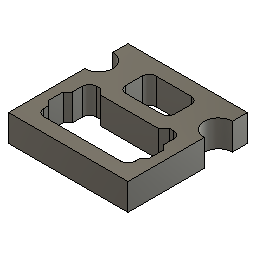
TinyNES_Foam_Top (Autodesk Fusion 360 design; units mm, degrees)
Autodesk Fusion 360 part; units mm, degrees
sketch "Sketch1" plane through (0, 0, 0) normal (0, 1, 0) x (1, 0, 0)
  line L0 (0, 0) -> (170, 0)
  line L1 (170, 0) -> (170, 170)
  line L2 (170, 170) -> (0, 170)
  line L3 (0, 170) -> (0, 0)
  line L4 (85, 170) -> (85, 128.5) construction
  line L5 (110, 107) -> (60, 107)
  line L6 (50, 117) -> (50, 140)
  line L7 (60, 150) -> (110, 150)
  line L8 (120, 140) -> (120, 117)
  line L9 (120, 107) -> (50, 150) construction
  line L10 (50, 107) -> (120, 150) construction
  arc A0 (60, 150) -> (50, 140) centre (60, 140) ccw
  arc A1 (120, 140) -> (110, 150) centre (110, 140) ccw
  arc A2 (110, 107) -> (120, 117) centre (110, 117) ccw
  arc A3 (50, 117) -> (60, 107) centre (60, 117) ccw
  line L11 (85, 128.5) -> (0, 128.5) construction
  line L12 (85, 128.5) -> (170, 128.5) construction
  arc A4 (0, 108.5) -> (0, 148.5) centre (0, 128.5) ccw
  arc A5 (170, 148.5) -> (170, 108.5) centre (170, 128.5) ccw
  line L13 (85, 0) -> (85, 53.5) construction
  line L14 (140, 20) -> (30, 20)
  line L15 (20, 30) -> (20, 87)
  line L16 (150, 87) -> (150, 30)
  line L17 (150, 20) -> (20, 87) construction
  line L18 (20, 20) -> (150, 87) construction
  arc A6 (20, 30) -> (30, 20) centre (30, 30) ccw
  arc A7 (140, 20) -> (150, 30) centre (140, 30) ccw
  line L19 (85, 53.5) -> (20, 53.5) construction
  line L20 (85, 53.5) -> (150, 53.5) construction
  line L21 (20, 53.5) -> (13.5, 53.5) construction
  line L22 (13.5, 53.5) -> (13.5, 64)
  line L23 (13.5, 53.5) -> (13.5, 43)
  line L24 (13.5, 43) -> (13.5, 36.5) construction
  line L25 (13.5, 36.5) -> (20, 36.5) construction
  line L26 (13.5, 64) -> (13.5, 70.5) construction
  line L27 (13.5, 70.5) -> (20, 70.5) construction
  line L28 (13.5, 64) -> (20, 70.5)
  line L29 (13.5, 43) -> (20, 36.5)
  line L30 (156.5, 64) -> (150, 70.5)
  line L31 (156.5, 53.5) -> (156.5, 64)
  line L32 (156.5, 53.5) -> (156.5, 43)
  line L33 (156.5, 43) -> (150, 36.5)
  line L34 (85, 53.5) -> (85, 87) construction
  line L35 (85, 128.5) -> (85, 87) construction
  line L36 (85, 87) -> (43.25, 87)
  line L37 (43.25, 87) -> (35.25, 95)
  line L38 (30, 95) -> (35.25, 95)
  line L39 (35.25, 95) -> (35.25, 87) construction
  line L40 (35.25, 87) -> (43.25, 87) construction
  line L41 (30, 95) -> (30, 85) construction
  arc A8 (30, 95) -> (20, 85) centre (30, 85) ccw
  line L42 (30, 85) -> (30, 95) construction
  line L43 (30, 85) -> (20, 85) construction
  arc A9 (150, 85) -> (140, 95) centre (140, 85) ccw
  line L44 (140, 95) -> (134.75, 95)
  line L45 (126.75, 87) -> (134.75, 95)
  line L46 (85, 87) -> (126.75, 87)
  point P0 (85, 128.5)
  point P1 (85, 53.5)
  dimension "d1" = 170
  dimension "d2" = 170
  dimension "d19" = 41.5
  dimension "d20" = 70
  dimension "d21" = 43
  dimension "d22" = 10
  dimension "d23" = 10
  dimension "d24" = 10
  dimension "d25" = 10
  dimension "d26" = 20
  dimension "d27" = 20
  dimension "d28" = 53.5
  dimension "d29" = 130
  dimension "d30" = 67
  dimension "d31" = 10
  dimension "d32" = 10
  dimension "d33" = 6.5
  dimension "d34" = 10.5
  dimension "d35" = 10.5
  dimension "d36" = 6.5
  dimension "d37" = 6.5
  dimension "d41" = 41.5
  dimension "d42" = 33.5
  dimension "d44" = 41.75
  dimension "d48" = 5.25
  dimension "d49" = 135
  dimension "d50" = 8
  dimension "d51" = 10
  dimension "d52" = 90
  dimension "d53" = 135
  dimension "d54" = 8
  constraint horizontal L0
  constraint vertical L1
  constraint horizontal L2
  constraint vertical L3
  constraint coincident L0.start L3.end
  constraint midpoint L2 L4.start
  constraint perpendicular L2 L4
  constraint horizontal L5
  constraint perpendicular L5 L6
  constraint parallel L5 L7
  constraint parallel L6 L8
  constraint coincident L9 P0
  constraint coincident L10 P0
  constraint coincident P0 L4.end
  constraint coincident L9.end L6
  constraint coincident L9.end L7
  constraint tangent L6 A0
  constraint tangent L7 A0
  constraint coincident L10.end L7
  constraint coincident L10.end L8
  constraint tangent L7 A1
  constraint tangent L8 A1
  constraint coincident L9.start L8
  constraint coincident L9.start L5
  constraint tangent L8 A2
  constraint tangent L5 A2
  constraint coincident L10.start L6
  constraint coincident L10.start L5
  constraint tangent L6 A3
  constraint tangent L5 A3
  constraint coincident L3 L11.end
  constraint perpendicular L3 L11
  constraint coincident L1 L12.end
  constraint perpendicular L1 L12
  constraint coincident L11.end A4.centre
  constraint coincident L12.end A5.centre
  constraint midpoint L0 L13.start
  constraint perpendicular L0 L13
  constraint horizontal L14
  constraint perpendicular L14 L15
  constraint parallel L15 L16
  constraint coincident L17 P1
  constraint coincident L18 P1
  constraint coincident P1 L13.end
  constraint coincident L18.start L15
  constraint coincident L18.start L14
  constraint tangent L15 A6
  constraint tangent L14 A6
  constraint coincident L17.start L14
  constraint coincident L17.start L16
  constraint tangent L14 A7
  constraint tangent L16 A7
  constraint coincident L15 L19.end
  constraint perpendicular L15 L19
  constraint coincident L16 L20.end
  constraint perpendicular L16 L20
  constraint perpendicular L15 L21
  constraint perpendicular L21 L22
  constraint perpendicular L21 L23
  constraint parallel L23 L24
  constraint coincident L15 L25.end
  constraint perpendicular L15 L25
  constraint perpendicular L21 L26
  constraint coincident L15 L27.end
  constraint perpendicular L15 L27
  constraint symmetric L13 L21.end L31.start
  constraint symmetric L13 L22.end L30.start
  constraint symmetric L13 L23.end L32.end
  constraint symmetric L13 L25.end L33.end
  constraint symmetric L13 L27.end L30.end
  constraint equal L17 L18
  constraint perpendicular L34 L36
  constraint coincident L37 L38.end
  constraint coincident L37.end L38.end
  constraint horizontal L40
  constraint perpendicular L38 L41
  constraint coincident L41.end A8.centre
  constraint vertical L39
  constraint symmetric L38.start L34 A9.end
  constraint symmetric L35.end L34 L36.start
  constraint symmetric L34 L36.end L45.start
  constraint symmetric L34 L37.end L44.end
  constraint symmetric L34 A8.end A9.start
  constraint symmetric L34 A8 A9
  measures "d1" distance of L0.start L0.end
  measures "d2" distance of L0.start L2.end
  measures "d19" distance of L4.start P0
  measures "d20" distance of L9.end L10.end
  measures "d21" distance of L10.start L9.end
  measures "d22" radius of A0
  measures "d23" radius of A1
  measures "d24" radius of A2
  measures "d25" radius of A3
  measures "d26" radius of A4
  measures "d27" radius of A5
  measures "d28" distance of L13.start P1
  measures "d29" distance of L15.end L16.start
  measures "d30" distance of L18.start L15.end
  measures "d31" radius of A6
  measures "d32" radius of A7
  measures "d33" distance of L19.end L21.end
  measures "d34" distance of L21.end L22.end
  measures "d35" distance of L21.end L23.end
  measures "d36" distance of L23.end L24.end
  measures "d37" distance of L22.end L26.end
  measures "d41" distance of L34.end P0
  measures "d42" distance of P1 L34.end
  measures "d44" distance of L34.end L36.end
  measures "d48" distance of L38.start L37.end
  measures "d49" angle of L37 L38
  measures "d50" distance of L37.end L39.end
  measures "d51" distance of L38.start L41.end
  measures "d52" angle of L42 L43
  measures "d53" angle of L36 L37
  measures "d54" distance of L36.end L39.end
extrude "Extrude1" add sketch "Sketch1" along normal blind 38.1 contours L0 L1 L2 L3 A4 A5
